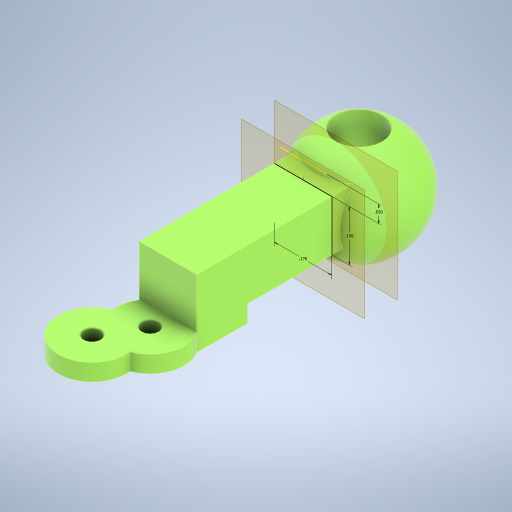
# Autodesk Inventor part: Left Arm
Saved by Autodesk Inventor 2023 (Build 270158000, 158)
## iProperties
Created: 2022-05-02
Part Number: Left Arm
Material: Phenolic Resin
Document SubType Name: Modeling
Designer: Devin
Density: 1.38 g/cm^3
Appearance: Light Green
Author: Devin
Autodesk Inventor part; units mm, degrees
ref_plane "YZ Plane" through (0, 0, 0) normal (1, 0, 0) x (0, 1, 0)
ref_plane "XZ Plane" through (0, 0, 0) normal (0, 1, 0) x (-1, 0, 0)
sketch "Sketch1" plane through (0, 0, 0) normal (0, 0, 1) x (1, 0, 0)
  line L0 (0, 3.81) -> (1.746, 3.81)
  line L1 (0, 0) -> (0, 7.4896) construction
  line L2 (0, 0) -> (13.1944, 0) construction
  line L3 (0, -3.81) -> (1.746, -3.81)
  arc A0 (1.746, -3.81) -> (1.746, 3.81) centre (0, 0) ccw
  line L4 (0, 3.81) -> (0, -3.81)
  point P0 (-6.8886, 3.81)
  point P1 (6.6767, 3.81)
  point P2 (0, 4.191)
  point P3 (0, 4.191)
  point P4 (-6.8886, -3.81)
  point P5 (6.6767, -3.81)
  point P6 (0, 4.191)
  point P7 (4.191, 0)
  dimension "d1" = 0.381
  dimension "d11" = 4.191
  constraints: 10 end point, 3 coincident, 3 point on circle, 3 point on line, 2 horizontal, 2 symmetric about line, 2 vertical, 1 centre point, 1 vertical alignment
  measures "d1" distance from line of point (0, 4.191) L0
  measures "d11" distance from line of point (4.191, 0) L4
revolve "Revolution1" add sketch "Sketch1" angle 360 about axis through (0, 0, 0) along (0, 1, 0)
sketch "Sketch2" plane through (0, 3.81, 0) normal (0, 1, 0) x (1, 0, 0)
  circle A0 centre (0, 0) radius 1.746 projected
  dimension "d3" = 3.4919
  constraints: 1 coincident
  measures "d3" diameter of A0
hole "Hole1" at (0, 3.81, 0) direction (0, -1, 0) diameter 3.4798 end through all
ref_plane "Work Plane1" through (0, 0, 4.191) normal (0, 0, 1) x (1, 0, 0)
sketch "Sketch3" plane through (0, 0, 4.191) normal (0, 0, 1) x (1, 0, 0)
  line L0 (-2.159, 2.54) -> (2.159, 2.54)
  line L1 (2.159, 2.54) -> (2.159, -1.27)
  line L2 (2.159, -1.27) -> (-2.159, -1.27)
  line L3 (-2.159, -1.27) -> (-2.159, 2.54)
  line L4 (1.746, 3.81) -> (-1.746, 3.81) projected
  point P0 (0, 0)
  point P1 (0, 2.54)
  dimension "d13" = 4.318
  dimension "d14" = 3.81
  dimension "d15" = 1.27
  constraints: 8 end point, 2 parallel, 1 horizontal, 1 midpoint, 1 perpendicular, 1 vertical alignment
  measures "d13" distance of L1.end L2.end
  measures "d14" distance of L0.end L1.end
  measures "d15" distance between parallel lines of L4 L0
extrude "Extrusion1" add sketch "Sketch3" along normal blind 10.16
ref_plane "Work Plane2" through (0, 0, 1.7399) normal (0, 0, 1) x (1, 0, 0)
extrude "Extrusion2" add sketch "Sketch3" against normal up to surface (2.4511 mm away)
sketch "Sketch4" plane through (0, -1.27, 0) normal (0, -1, 0) x (1, 0, 0)
  line L0 (2.159, 2.54) -> (2.159, 14.351) projected
  line L1 (2.159, 10.541) -> (-2.159, 10.541)
  line L2 (-2.159, 10.541) -> (-2.159, 14.351)
  line L3 (-2.159, 14.351) -> (2.159, 14.351)
  line L4 (2.159, 14.351) -> (2.159, 10.541) construction
  line L5 (-2.159, 14.351) -> (2.159, 14.351) projected
  circle A0 centre (0, 15.689) radius 0.635
  circle A1 centre (0, 15.689) radius 2.54
  circle A2 centre (-1.651, 18.401) radius 0.635
  circle A3 centre (-1.651, 18.401) radius 2.54
  point P0 (0, 0)
  point P1 (2.159, 14.351)
  point P2 (0, 14.351)
  point P3 (2.159, 14.351)
  point P4 (0.889, 18.401)
  point P5 (-2.5191, 16.014)
  point P6 (-1.3208, 17.8586)
  point P7 (0.8681, 18.0761)
  dimension "d31" = 5.08
  dimension "d22" = 3.81
  dimension "d25" = 1.27
  dimension "d27" = 5.08
  dimension "d30" = 1.27
  dimension "d32" = 1.27
  dimension "d33" = 4.318
  constraints: 8 end point, 4 point on line, 3 centre point, 3 coincident, 2 parallel, 2 point on circle, 1 horizontal, 1 horizontal alignment, 1 midpoint, 1 perpendicular, 1 tangent, 1 vertical alignment, 3 other
  measures "d22" distance between parallel lines of L5 L1
  measures "d25" diameter of A0
  measures "d27" diameter of A1
  measures "d30" diameter of A2
  measures "d32" distance from line of L0 point (0.889, 18.401)
  measures "d33" distance of L1.start L1.end
extrude "Extrusion4" add sketch "Sketch4" along normal blind 1.27
body "Solid1"
